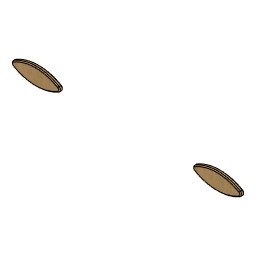
Lamello Bisquit Size10 Edge EDGE (Autodesk Fusion 360 design; units mm, degrees)
description: Lamello Bisquit
part number: Lamello Bisquit
Autodesk Fusion 360 part; units mm, degrees
sketch "ContactArea" plane through (0, 0, 0) normal (0, 0, 1) x (1, 0, 0)
  line L0 (-160, -12.5) -> (160, -12.5)
  line L1 (160, -12.5) -> (160, 12.5)
  line L2 (160, 12.5) -> (-160, 12.5)
  line L3 (-160, 12.5) -> (-160, -12.5)
  line L4 (-160, -12.5) -> (160, 12.5) construction
  line L5 (160, -12.5) -> (-160, 12.5) construction
  dimension "d4" = 25
  dimension "d5" = 320
  constraint horizontal L0
  constraint perpendicular L0 L1
  constraint parallel L0 L2
  constraint parallel L1 L3
  constraint coincident L4 origin
  constraint coincident L5 origin
  measures "d4" distance of L0.end L1.end
  measures "d5" distance of L1 L3
sketch "BoardCalc" plane through (0, 0, 0) normal (1, 0, 0) x (0, 1, 0)
  line L0 (0, 0) -> (-102, 0)
  line L1 (-102, 0) -> (-102, 18)
  line L2 (-102, 18) -> (18, 18)
  line L3 (18, 18) -> (0, 0)
  line L4 (18, 18) -> (18, -102)
  line L5 (18, -102) -> (0, -102)
  line L6 (0, -102) -> (0, 0)
  line L7 (-7.4781, 12.3209) -> (-3.5183, 16.2807)
  line L8 (-0.902, 16.7756) -> (16.7756, -0.902)
  line L9 (16.2807, -3.5183) -> (12.3209, -7.4781)
  line L10 (9.7046, -7.9731) -> (-7.9731, 9.7046)
  line L11 (-5.4982, 14.3008) -> (14.3008, -5.4982) construction
  line L12 (-3.5183, 16.2807) -> (-0.902, 16.7756)
  line L13 (-7.4781, 12.3209) -> (-7.9731, 9.7046)
  line L14 (16.7756, -0.902) -> (16.2807, -3.5183)
  line L15 (12.3209, -7.4781) -> (9.7046, -7.9731)
  line L16 (7.9368, 7.9368) -> (0.8657, 0.8657) construction
  line L17 (0, 0) -> (0.8657, 0.8657) construction
  line L18 (-0.902, 16.7756) -> (-0.902, 18) construction
  line L19 (-260, 70) -> (-279.2315, 70) construction
  line L20 (-293.1122, 66.8878) -> (-286.8878, 66.8878) construction
  point P0 (-9.0337, 10.7652)
  point P1 (-1.9627, 17.8363)
  point P2 (17.8363, -1.9627)
  point P3 (10.7652, -9.0337)
  dimension "d7" = 18
  dimension "d8" = 120
  dimension "d9" = 90
  dimension "d10" = 120
  dimension "d12" = 18
  dimension "d13" = 10
  dimension "d14" = 28
  dimension "d15" = 2.2
  dimension "d16" = 1.5
  dimension "d17" = 2.2
  dimension "d18" = 1.5
  dimension "d19" = 1.5
  dimension "d20" = 2.2
  dimension "d21" = 2.2
  dimension "d22" = 1.5
  dimension "EdgeEdgeOtherSideRefYCoordinateDriven" = 19.2315
  dimension "EdgeEdgeReferenceCoordDriven" = 6.2244
  dimension "d30" = 19.2315
  dimension "d31" = 6.2244
  constraint coincident L0.start L3.end
  constraint horizontal L0
  constraint perpendicular L0 L1
  constraint perpendicular L1 L2
  constraint parallel L4 L6
  constraint perpendicular L5 L6
  constraint perpendicular L7 L8
  constraint parallel L7 L9
  constraint parallel L8 L10
  constraint coincident L7 L11.start
  constraint coincident P1 L7
  constraint coincident P1 L8
  constraint coincident P0 L7
  constraint coincident P0 L10
  constraint coincident L9 L11.end
  constraint coincident P2 L8
  constraint coincident P2 L9
  constraint coincident P3 L9
  constraint coincident P3 L10
  constraint midpoint L7 L11.start
  constraint midpoint L9 L11.end
  constraint midpoint L8 L16.start
  constraint midpoint L10 L16.end
  constraint collinear L3 L16
  constraint coincident L2 L18.end
  constraint perpendicular L2 L18
  constraint equal L17 L18
  measures "d7" distance of L0 L2
  measures "d8" distance of L1 L2.end
  measures "d9" angle of L0 L6
  measures "d10" distance of L2 L5.end
  measures "d12" distance of L4 L5.end
  measures "d13" distance of L8 L10
  measures "d14" distance of L7 L9
  measures "d15" distance of P1 L7.end
  measures "d16" distance of P1 L8.start
  measures "d17" distance of P0 L7.start
  measures "d18" distance of P0 L10.end
  measures "d19" distance of P2 L8.end
  measures "d20" distance of P2 L9.start
  measures "d21" distance of P3 L9.end
  measures "d22" distance of P3 L10.start
  measures "EdgeEdgeOtherSideRefYCoordinateDriven" distance of L2.end L11
  measures "EdgeEdgeReferenceCoordDriven" distance of L0.start L11
  measures "d30" distance of L19.start L19.end
  measures "d31" distance of L20.start L20.end
sketch "Pin Postion" plane through (0, 0, 0) normal (0, 0, 1) x (1, 0, 0)
  circle A0 centre (100, 6.2756) radius 0.5
  line L0 (160, -12.5) -> (160, 12.5)
  line L1 (160, 12.5) -> (-160, 12.5)
  line L2 (0, -260) -> (0, -279.2315)
  line L3 (0, -293.1122) -> (0, -286.8878)
  point P0 (0, -260)
  point P1 (0, -279.2315)
  point P2 (0, -286.8878)
  point P3 (0, -293.1122)
  dimension "d32" = 1
  dimension "d36" = 60
  dimension "EdgeEdgeOtherSideRefYCoordinateDrivenProjected" = 19.2315
  dimension "EdgeEdgeRefCoordDrivenProjected" = 6.2244
  dimension "d48" = 6.2244
  measures "d32" diameter of A0
  measures "d36" distance of A0.centre L0
  measures "EdgeEdgeOtherSideRefYCoordinateDrivenProjected" distance of P0 P1
  measures "EdgeEdgeRefCoordDrivenProjected" distance of P2 P3
  measures "d48" distance of A0.centre L1
extrude "Extrude1" add sketch "Pin Postion" along normal blind 10 makes body 1
pattern_linear "R-Pattern1" count 2 spacing 200 along (-1, 0, 0) of bodies 1 makes body 2
sketch "Sketch1" plane through (0, 0, 0) normal (0, 0, 1) x (1, 0, 0) in component "Lamello v1"
  line L0 (31.5, -2) -> (-31.5, -2)
  line L1 (-31.5, -2) -> (-31.5, 2)
  line L2 (-31.5, 2) -> (31.5, 2)
  line L3 (31.5, 2) -> (31.5, -2)
  line L4 (31.5, -2) -> (-31.5, 2) construction
  line L5 (-31.5, -2) -> (31.5, 2) construction
  dimension "d8_1" = 4
  dimension "d9_1" = 63
  constraint horizontal L0
  constraint perpendicular L0 L1
  constraint parallel L0 L2
  constraint parallel L1 L3
  constraint coincident L4 origin
  constraint coincident L5 origin
  measures "d8_1" distance of L0 L2
  measures "d9_1" distance of L1 L3
extrude "Extrude1'" add sketch "Sketch1" along normal mid plane 20 separate body makes body 3 in component "Lamello v1"
sketch "Sketch2" plane through (0, 0, 0) normal (0, 1, 0) x (1, 0, 0) in component "Lamello v1"
  arc A0 (25.0416, 2.5736) -> (-25.0416, 2.5736) centre (0, -39.2308) ccw
  arc A1 (-25.0416, -2.5736) -> (25.0416, -2.5736) centre (0, 39.2308) ccw
  circle A2 centre (-23.5, 0) radius 3
  circle A3 centre (23.5, 0) radius 3
  point P0 (-26.5, 0)
  point P1 (26.5, 0)
  point P2 (0, 9.5)
  point P3 (0, -9.5)
  dimension "d12_1" = 6
  dimension "d13_1" = 6
  dimension "d14_1" = 53
  dimension "d15_1" = 19
  constraint vertical origin A1.centre
  constraint vertical origin A0.centre
  constraint vertical A0.end A1.start
  constraint vertical A0.start A1.end
  constraint horizontal origin A2.centre
  constraint coincident A0.end A2
  constraint coincident A1.start A2
  constraint tangent A0 A2
  constraint tangent A1 A2
  constraint horizontal origin A3.centre
  constraint coincident A0.start A3
  constraint tangent A0 A3
  constraint coincident A2 P0
  constraint coincident A3 P1
  constraint horizontal origin P0
  constraint horizontal origin P1
  constraint coincident A1 P3
  constraint vertical origin P2
  constraint vertical origin P3
  constraint coincident A0 P2
  measures "d12_1" diameter of A2
  measures "d13_1" diameter of A3
  measures "d14_1" distance of P0 P1
  measures "d15_1" distance of P2 P3
extrude "Extrude2" add sketch "Sketch2" along normal mid plane 4 separate body makes body 4 in component "Lamello v1"
fillet "Fillet1" radius 1 8 edges at (0, 2, -9.5) (-26.5, 2, 0) (0, 2, 9.5) (26.5, 2, 0) (0, -2, -9.5) (26.5, -2, 0) (0, -2, 9.5) (-26.5, -2, 0) on bodies 4 in component "Lamello v1"
sketch "Sketch3" plane through (0, 0, 0) normal (0, 0, 1) x (1, 0, 0) in component "Lamello v1"
pattern_linear "00000000-0000-0000-0000-000000000000" [suppressed]
component "Lamello v1" placed x (1, 0, 0) y (0, 1, 0) z (0, 0, 1) at (100, 6.2756, 0)
component "Lamello v1" placed x (1, 0, 0) y (0, 1, 0) z (0, 0, 1) at (-100, 6.2756, 0)
hidden bodies 1 2 3
equation "ContactPatchHeight = 25 mm"
equation "ContactPatchWidth = 320 mm"
equation "ConnectionAngle = 90 deg" comment "Only values from 20 deg to 180 deg are valid.Otherwise it will be calculations!"
equation "d4 = ContactPatchHeight"
equation "d5 = ContactPatchWidth"
equation "NestledBoardT = 18 mm" comment "Caclucated Automatically!"
equation "d7 = NestledBoardT"
equation "d9 = ConnectionAngle"
equation "PillarBoardT = 18 mm" comment "Calculated Automatically!"
equation "d12 = PillarBoardT"
equation "EdgeEdgeReferenceCoord = EdgeEdgeRefCoordDrivenProjected"
equation "EdgeEdgeOtherSideRefYCoordinate = EdgeEdgeOtherSideRefYCoordinateDrivenProjected"
equation "d30 = EdgeEdgeOtherSideRefYCoordinateDriven"
equation "d31 = EdgeEdgeReferenceCoordDriven"
equation "X_Coord = if(Count < 1; ( ContactPatchWidth / 2 ); DistFromSide1)"
equation "Y_Coord = EdgeEdgeReferenceCoord"
equation "Shift_Y = 0 mm"
equation "d36 = X_Coord"
equation "d37 = Y_Coord + Shift_Y"
equation "DistFromSide1 = 60 mm"
equation "DistFromSide2 = 60 mm"
equation "MinDistBetween = 96 mm"
equation "MaxDistBetween = 480 mm"
equation "PlacingWidth = ContactPatchWidth - DistFromSide1 - DistFromSide2"
equation "Count = if(MinDistBetween > PlacingWidth; 0; ceil(PlacingWidth / MaxDistBetween))"
equation "Step = PlacingWidth / Count"
equation "d48 = Y_Coord + Shift_Y"
equation "d51 = Count + 1"
equation "d53 = -Step"
equation "LamelloLength = 53 mm" comment "Size20 = 56mm; Size10 = 53 mm; Size0 = 47 mm; SizeH9 = 38 mm"
equation "LamelloWidth = 19 mm" comment "Size20 = 23mm; Size10 = 19mm; Size0 = 15 mm; SizeH9 =12 mm"
equation "LamelloThickness = 4 mm" comment "Size20 = 4mm; Size10 = 4 mm; Size0 = 4 mm; SizeH9 = 3mm"
equation "Tolerance = 1 mm" comment "Recommended tolerance for cutting"
equation "GrooveLength = LamelloLength + Tolerance + 9 mm"
equation "GrooveWidth = LamelloWidth + 1 mm"
equation "GrooveThickness = LamelloThickness"
equation "d8_1 = GrooveThickness"
equation "d9_1 = GrooveLength"
equation "d10_1 = GrooveWidth"
equation "d14_1 = LamelloLength"
equation "d15_1 = LamelloWidth"
equation "d16_1 = LamelloThickness"
equation "d71 = Count + 1"
equation "d73 = Step"
named bodies: "Lamello Hole", "Lamello"
